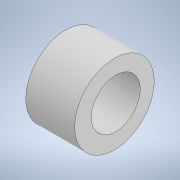
# Autodesk Inventor part: bushing
Saved by Autodesk Inventor 2021 (Build 250183000, 183)
## iProperties
Created: 2022-04-24
Part Number: bushing
Material: Generic
Document SubType Name: Modeling
Designer: hp
Density: 1 g/cm^3
Appearance: Default
Author: hp
Autodesk Inventor part; units mm, degrees
ref_plane "YZ Plane" through (0, 0, 0) normal (1, 0, 0) x (0, 1, 0)
ref_plane "XZ Plane" through (0, 0, 0) normal (0, 1, 0) x (-1, 0, 0)
ref_plane "XY Plane" through (0, 0, 0) normal (0, 0, 1) x (1, 0, 0)
sketch "Sketch1" plane through (0, 0, 0) normal (1, 0, 0) x (0, 1, 0)
  circle A0 centre (0, 0) radius 8
  circle A1 centre (0, 0.4361) radius 13
  dimension "d0" = 26
  dimension "d1" = 16
  constraints: 2 centre point, 1 coincident
  measures "d0" diameter of A1
  measures "d1" diameter of A0
extrude "Extrusion1" add sketch "Sketch1" along normal blind 16
body "Solid1"
